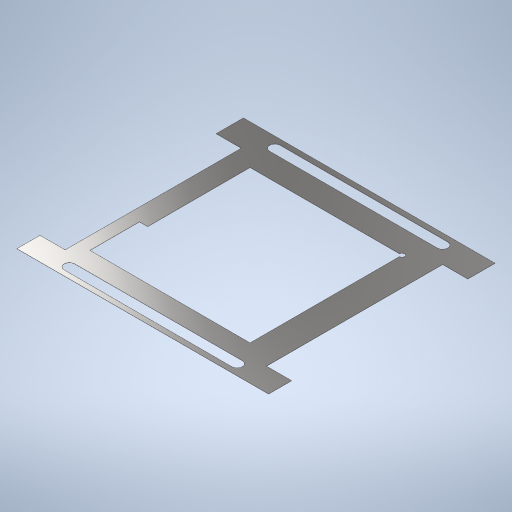
# Autodesk Inventor part: Baseplate Film Stencil - V1
Saved by Autodesk Inventor 2023 (Build 270158000, 158)
## iProperties
Created: 2022-06-23
Part Number: Baseplate Film Stencil - V1
Material: Stainless Steel
Document SubType Name: Modeling
Designer: Caleb
Density: 8 g/cm^3
Appearance: Semi-Polished
Author: Caleb
Autodesk Inventor part; units mm, degrees
ref_plane "YZ Plane" through (0, 0, 0) normal (1, 0, 0) x (0, 1, 0)
ref_plane "XZ Plane" through (0, 0, 0) normal (0, 1, 0) x (-1, 0, 0)
ref_plane "XY Plane" through (0, 0, 0) normal (0, 0, 1) x (1, 0, 0)
sketch "Sketch1" plane through (0, 0, 0) normal (0, 1, 0) x (-1, 0, 0)
  line L0 (-38.1, -34.29) -> (38.1, -34.29)
  line L1 (38.1, -34.29) -> (38.1, 34.29)
  line L2 (38.1, 34.29) -> (-38.1, 34.29)
  line L3 (-38.1, 34.29) -> (-38.1, -34.29)
  line L4 (-38.1, -34.29) -> (38.1, 34.29) construction
  line L5 (38.1, -34.29) -> (-38.1, 34.29) construction
  point P0 (0, 0)
  dimension "d0" = 76.2
  dimension "d1" = 68.58
  constraints: 12 end point, 2 midpoint, 2 parallel, 1 horizontal, 1 perpendicular
  measures "d0" distance of L2.end L1.end
  measures "d1" distance of L1.end L0.end
extrude "Extrusion1" add sketch "Sketch1" along normal blind 0.0508
sketch "Sketch2" plane through (0, 0.0508, 0) normal (0, 1, 0) x (1, 0, 0)
  line L0 (-38.1, -34.29) -> (38.1, -34.29) projected
  line L1 (-46.3971, 0) -> (43.7494, 0)
  line L2 (-38.1, 34.29) -> (-38.1, -34.29) projected
  line L3 (38.1, -34.29) -> (38.1, 34.29) projected
  line L4 (38.1, 26.035) -> (30.48, 26.035)
  line L5 (30.48, 26.035) -> (30.48, -27.305)
  line L6 (30.48, -27.305) -> (38.1, -27.305)
  line L7 (38.1, -27.305) -> (38.1, 26.035)
  line L8 (0, -45.6355) -> (0, 71.8702)
  line L9 (46.3971, 0) -> (-43.7494, 0)
  line L10 (-38.1, -34.29) -> (-38.1, 34.29)
  line L11 (-38.1, 26.035) -> (-30.48, 26.035)
  line L12 (-30.48, 26.035) -> (-30.48, -27.305)
  line L13 (-30.48, -27.305) -> (-38.1, -27.305)
  line L14 (-38.1, -27.305) -> (-38.1, 26.035)
  line L15 (38.1, 34.29) -> (-38.1, 34.29) projected
  point P0 (0, 0)
  point P1 (38.1, -27.305)
  point P2 (-38.1, -27.305)
  dimension "d13" = 53.34
  dimension "d14" = 7.62
  dimension "d16" = 8.255
  constraints: 24 end point, 6 symmetric about line, 2 horizontal, 2 parallel, 2 point on line, 1 perpendicular, 1 vertical
  measures "d13" distance of L4.end L5.end
  measures "d14" distance of L5.end L6.end
  measures "d16" distance between parallel lines of L15 L4
extrude "Extrusion2" cut sketch "Sketch2" against normal through all contours L2 L1 L12 L13 | L2 L11 L12 L1 | L6 L5 L1 L3 | L5 L4 L3 L1
sketch "Sketch3" plane through (0, 0.0508, 0) normal (0, 1, 0) x (1, 0, 0)
  line L0 (25.4, -31.115) -> (-25.4, -31.115) construction
  line L1 (25.4, -29.5275) -> (-25.4, -29.5275)
  line L2 (-25.4, -32.7025) -> (25.4, -32.7025)
  arc A0 (25.4, -32.7025) -> (25.4, -29.5275) centre (25.4, -31.115) ccw
  arc A1 (-25.4, -29.5275) -> (-25.4, -32.7025) centre (-25.4, -31.115) ccw
  line L3 (25.4, 31.115) -> (-25.4, 31.115) construction
  line L4 (25.4, 32.7025) -> (-25.4, 32.7025)
  line L5 (-25.4, 29.5275) -> (25.4, 29.5275)
  arc A2 (25.4, 29.5275) -> (25.4, 32.7025) centre (25.4, 31.115) ccw
  arc A3 (-25.4, 32.7025) -> (-25.4, 29.5275) centre (-25.4, 31.115) ccw
  line L6 (38.1, 34.29) -> (-38.1, 34.29) projected
  line L7 (-38.1, -34.29) -> (38.1, -34.29) projected
  point P0 (0, 0)
  point P1 (0, -31.115)
  point P2 (0, 31.115)
  dimension "d17" = 3.175
  dimension "d18" = 3.175
  dimension "d19" = 50.8
  dimension "d20" = 50.8
  dimension "d21" = 3.175
  dimension "d22" = 3.175
  constraints: 16 end point, 8 point on circle, 8 tangent, 4 centre point, 3 parallel, 2 midpoint, 2 vertical alignment, 1 horizontal
  measures "d17" distance between parallel lines of L2 L1
  measures "d18" distance between parallel lines of L4 L5
  measures "d19" distance of L0.end L0.start
  measures "d20" distance of L3.end L3.start
  measures "d21" distance from line of L6 point (0, 31.115)
  measures "d22" distance from line of L7 point (0, -31.115)
extrude "Extrusion3" cut sketch "Sketch3" against normal through all
sketch "Sketch4" plane through (0, 0.0508, 0) normal (0, 1, 0) x (1, 0, 0)
  line L0 (-24.105, -23.69) -> (21.895, -23.69)
  line L1 (21.895, -23.69) -> (21.895, 22.31)
  line L2 (21.895, 22.31) -> (-24.105, 22.31)
  line L3 (-24.105, 22.31) -> (-24.105, -23.69)
  line L4 (38.1, 34.29) -> (-38.1, 34.29) projected
  line L5 (38.1, 26.035) -> (38.1, 34.29) projected
  circle A0 centre (21.895, 22.31) radius 0.7938
  line L6 (29.845, -22.86) -> (-29.845, -22.86) construction
  line L7 (-29.845, -22.86) -> (-29.845, 22.86) construction
  line L8 (-29.845, 22.86) -> (29.845, 22.86) construction
  line L9 (29.845, 22.86) -> (29.845, -22.86) construction
  line L10 (29.845, -22.86) -> (-29.845, 22.86) construction
  line L11 (-29.845, -22.86) -> (29.845, 22.86) construction
  point P0 (0, 0)
  point P1 (21.895, 21.5163)
  point P2 (21.1012, 22.31)
  dimension "d29" = 1.5875
  dimension "d30" = 59.69
  dimension "d31" = 45.72
  dimension "d32" = 7.95
  dimension "d33" = 0.55
  dimension "d34" = 46
  dimension "d35" = 46
  constraints: 20 end point, 4 parallel, 2 horizontal, 2 midpoint, 2 perpendicular, 1 centre point, 1 coincident
  measures "d29" diameter of A0
  measures "d30" distance of L6.start L6.end
  measures "d31" distance of L6.end L7.end
  measures "d32" distance between parallel lines of L9 L1
  measures "d33" distance between parallel lines of L8 L2
  measures "d34" distance of L0.start L0.end
  measures "d35" distance of L2.end L0.start
extrude "Extrusion4" cut sketch "Sketch4" against normal through all
sketch "Sketch5" plane through (0, 0.0508, 0) normal (0, 1, 0) x (1, 0, 0)
  line L0 (-24.105, -23.69) -> (-24.105, 22.31) projected
  line L1 (-24.105, -23.69) -> (-26.605, -23.69)
  line L2 (-26.605, -23.69) -> (-26.605, -8.69)
  line L3 (-26.605, -8.69) -> (-24.105, -8.69)
  line L4 (-24.105, -8.69) -> (-24.105, -23.69)
  point P0 (0, 0)
  dimension "d36" = 15
  dimension "d37" = 2.5
  constraints: 8 end point, 2 parallel, 1 horizontal, 1 perpendicular
  measures "d36" distance of L1.end L2.end
  measures "d37" distance of L2.end L3.end
extrude "Extrusion5" cut sketch "Sketch5" against normal through all
equation "\"d18\" = d17"
equation "\"d20\" = d19"
body "Solid1"
